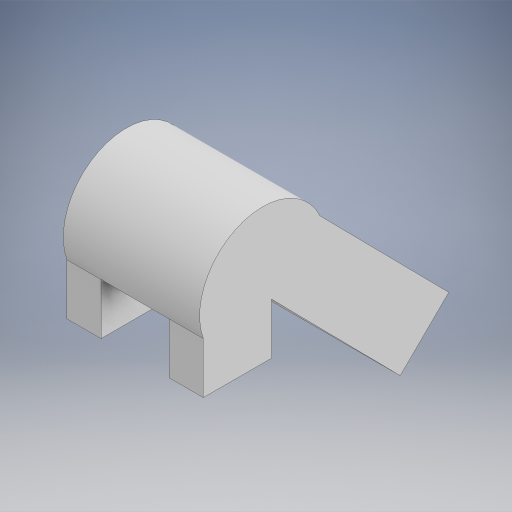
# Autodesk Inventor part: hook2
Saved by Autodesk Inventor 2024.2 (Build 282272000, 272)
## iProperties
Created: 2024-03-09
Part Number: hook2
Material: Generic
Document SubType Name: Modeling
Designer: rohan
Density: 1 g/cm^3
Appearance: Default
Author: rohan
Autodesk Inventor part; units mm, degrees
ref_plane "YZ Plane" through (0, 0, 0) normal (1, 0, 0) x (0, 1, 0)
ref_plane "XZ Plane" through (0, 0, 0) normal (0, 1, 0) x (-1, 0, 0)
ref_plane "XY Plane" through (0, 0, 0) normal (0, 0, 1) x (1, 0, 0)
sketch "Sketch1" plane through (0, 0, 0) normal (1, 0, 0) x (0, 1, 0)
  line L0 (29.5838, 2.29) -> (48.6338, 2.29)
  line L1 (48.6338, 2.29) -> (48.6338, -23.11)
  line L2 (48.6338, -23.11) -> (29.5838, -23.11)
  line L3 (29.5838, -23.11) -> (29.5838, 2.29)
  line L4 (48.6338, -23.11) -> (0, -71.0648)
  line L5 (0, -71.0648) -> (17.8338, -89.1511)
  line L6 (17.8338, -89.1511) -> (66.4676, -41.1964)
  line L7 (66.4676, -41.1964) -> (48.6338, -23.11)
  arc A0 (66.4676, -41.1964) -> (48.6338, 2.29) centre (56.5947, -19.8453) ccw
  point P0 (0, 0)
  dimension "d0" = 19.05
  dimension "d1" = 25.4
  dimension "d2" = 25.4
  constraints: 16 end point, 4 parallel, 2 perpendicular, 2 point on circle, 1 centre point, 1 horizontal
  measures "d0" distance of L1.end L2.end
  measures "d1" distance of L0.end L1.end
  measures "d2" distance of L5.end L4.end
extrude "Extrusion1" add sketch "Sketch1" along normal blind 12.7
ref_plane "Work Plane1" through (25.4, 0, 0) normal (1, 0, 0) x (0, 0, -1)
mirror "Mirror1" about plane through (25.4, 0, 0) normal (1, 0, 0) of "Extrusion1"
sketch "Sketch2" plane through (12.7, 0, 0) normal (1, 0, 0) x (0, 0, -1)
  line L0 (23.11, 48.6338) -> (71.0648, 0) projected
  line L1 (23.11, 48.6338) -> (-2.29, 48.6338)
  arc A0 (41.1964, 66.4676) -> (-2.29, 48.6338) centre (19.8453, 56.5947) ccw projected
  line L2 (89.1511, 17.8338) -> (41.1964, 66.4676) projected
  line L3 (71.0648, 0) -> (89.1511, 17.8338) projected
  point P0 (0, 0)
  constraints: 2 end point, 1 point on circle
extrude "Extrusion2" add sketch "Sketch2" along normal up to surface (25.4 mm away)
body "Solid1"
